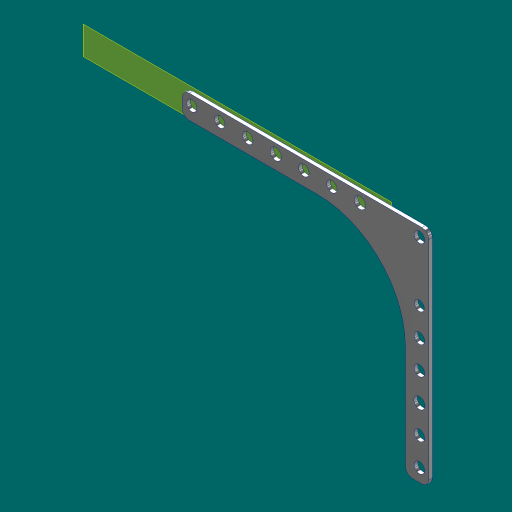
# Autodesk Inventor part: UnderGusset
Saved by Autodesk Inventor 2023.1 (Build 271208000, 208)
## iProperties
Created: 2022-11-06
Part Number: UnderGusset
Material: Aluminum 6061
Document SubType Name: Modeling
Designer: zac-h
Density: 2.7 g/cm^3
Appearance: Aluminum - Flat
Author: zac-h
Autodesk Inventor part; units mm, degrees
ref_plane "YZ Plane" through (0, 0, 0) normal (1, 0, 0) x (0, 1, 0)
ref_plane "XZ Plane" through (0, 0, 0) normal (0, 1, 0) x (-1, 0, 0)
ref_plane "XY Plane" through (0, 0, 0) normal (0, 0, 1) x (1, 0, 0)
ref_plane "Work Plane1" through (0, 0, 0) normal (0, 0, 1) x (1, 0, 0)
sketch "Sketch1" plane through (0, 0, 0) normal (0, 0, 1) x (1, 0, 0)
  line L0 (468.9048, -89.2586) -> (468.9048, 5.0009) projected
  arc A0 (468.9048, 5.0009) -> (465.7298, 8.1759) centre (465.7298, 5.0009) ccw projected
  line L1 (465.7298, 8.1759) -> (360.311, 8.1759) projected
  line L2 (458.2368, -92.4336) -> (458.2368, -2.4921)
  line L3 (458.2368, -2.4921) -> (357.136, -2.4921)
  arc A1 (360.311, 8.1759) -> (357.136, 5.0009) centre (360.311, 5.0009) ccw projected
  line L4 (357.136, 5.0009) -> (357.136, -89.2586) projected
  arc A2 (357.136, -89.2586) -> (360.311, -92.4336) centre (360.311, -89.2586) ccw projected
  line L5 (360.311, -92.4336) -> (465.7298, -92.4336) projected
  arc A3 (465.7298, -92.4336) -> (468.9048, -89.2586) centre (465.7298, -89.2586) ccw projected
  line L6 (468.9048, -89.2586) -> (468.9048, 5.0009) projected
  arc A4 (468.9048, 5.0009) -> (465.7298, 8.1759) centre (465.7298, 5.0009) ccw projected
  line L7 (465.7298, 8.1759) -> (360.311, 8.1759) projected
  circle A5 centre (437.65, 3.8619) radius 2.5844 projected
  circle A6 centre (372.6092, -23.0789) radius 2.5844 projected
  circle A7 centre (399.55, -88.1196) radius 2.5844 projected
  circle A8 centre (464.5908, -61.1789) radius 2.5844 projected
  circle A9 centre (372.6092, -88.1196) radius 2.413 projected
  circle A10 centre (412.25, 3.8619) radius 2.413 projected
  circle A11 centre (464.5908, -73.8789) radius 2.413 projected
  circle A12 centre (464.5908, -48.4789) radius 2.413 projected
  circle A13 centre (464.5908, -35.7789) radius 2.413 projected
  circle A14 centre (374.15, 3.8619) radius 2.413 projected
  circle A15 centre (386.85, 3.8619) radius 2.413 projected
  arc A16 (365.5823, -19.7251) -> (365.5823, -17.8759) centre (362.2803, -18.8005) ccw projected
  line L8 (365.5823, -19.7251) -> (365.5823, -22.1025) projected
  line L9 (365.5823, -22.1025) -> (363.2049, -22.1025) projected
  arc A17 (361.3557, -22.1025) -> (363.2049, -22.1025) centre (362.2803, -18.8005) ccw projected
  line L10 (361.3557, -22.1025) -> (358.9783, -22.1025) projected
  line L11 (358.9783, -22.1025) -> (358.9783, -19.7251) projected
  arc A18 (358.9783, -17.8759) -> (358.9783, -19.7251) centre (362.2803, -18.8005) ccw projected
  line L12 (358.9783, -17.8759) -> (358.9783, -15.4985) projected
  line L13 (358.9783, -15.4985) -> (361.3557, -15.4985) projected
  arc A19 (363.2049, -15.4985) -> (361.3557, -15.4985) centre (362.2803, -18.8005) ccw projected
  line L14 (363.2049, -15.4985) -> (365.5823, -15.4985) projected
  line L15 (365.5823, -15.4985) -> (365.5823, -17.8759) projected
  circle A20 centre (424.95, 3.8619) radius 2.413 projected
  arc A21 (358.9783, -64.5327) -> (358.9783, -66.3818) centre (362.2803, -65.4572) ccw projected
  line L16 (358.9783, -64.5327) -> (358.9783, -62.1552) projected
  line L17 (358.9783, -62.1552) -> (361.3557, -62.1552) projected
  arc A22 (363.2049, -62.1552) -> (361.3557, -62.1552) centre (362.2803, -65.4572) ccw projected
  line L18 (363.2049, -62.1552) -> (365.5823, -62.1552) projected
  line L19 (365.5823, -62.1552) -> (365.5823, -64.5327) projected
  arc A23 (365.5823, -66.3818) -> (365.5823, -64.5327) centre (362.2803, -65.4572) ccw projected
  line L20 (365.5823, -66.3818) -> (365.5823, -68.7592) projected
  line L21 (365.5823, -68.7592) -> (363.2049, -68.7592) projected
  arc A24 (361.3557, -68.7592) -> (363.2049, -68.7592) centre (362.2803, -65.4572) ccw projected
  line L22 (361.3557, -68.7592) -> (358.9783, -68.7592) projected
  line L23 (358.9783, -68.7592) -> (358.9783, -66.3818) projected
  circle A25 centre (464.5908, -86.5789) radius 2.413 projected
  circle A26 centre (464.5908, -23.0789) radius 1.9844 projected
  circle A27 centre (464.5908, 3.8619) radius 2.413 projected
  circle A28 centre (361.45, 3.8619) radius 2.413 projected
  circle A29 centre (418.6, -42.1289) radius 36.6 projected
  circle A30 centre (437.65, -88.1196) radius 2.5844 projected
  circle A31 centre (372.6092, -61.1789) radius 2.5844 projected
  circle A32 centre (399.55, 3.8619) radius 2.5844 projected
  circle A33 centre (418.6, -42.1289) radius 39.6368
  circle A34 centre (464.5908, 3.8619) radius 2.2479
  circle A35 centre (464.5908, -23.0789) radius 2.2479
  circle A36 centre (464.5908, -35.7789) radius 2.2479
  circle A37 centre (464.5908, -48.4789) radius 2.2479
  circle A38 centre (464.5908, -61.1789) radius 2.2479
  circle A39 centre (464.5908, -73.8789) radius 2.2479
  circle A40 centre (464.5908, -86.5789) radius 2.2479
  circle A41 centre (437.65, 3.8619) radius 2.2479
  circle A42 centre (424.95, 3.8619) radius 2.2479
  circle A43 centre (412.25, 3.8619) radius 2.2479
  circle A44 centre (399.55, 3.8619) radius 2.2479
  circle A45 centre (386.85, 3.8619) radius 2.2479
  circle A46 centre (374.15, 3.8619) radius 2.2479
  circle A47 centre (361.45, 3.8619) radius 2.2479
  point P0 (0, 0)
  point P1 (418.6, -2.4921)
  point P2 (458.2368, -42.1289)
  dimension "d0" = 10.668
  dimension "d2" = 4.4958
  dimension "d5" = 12.7
  dimension "d10" = 4.4958
  dimension "d13" = 12.7
  constraints: 15 centre point, 4 coincident, 4 end point, 2 point on line, 1 equal radius, 1 horizontal, 1 perpendicular, 1 tangent, 1 vertical, 23 other
  measures "d0" distance between parallel lines of L0 L2
  measures "d2" diameter of A34
  measures "d5" distance of A35.centre A36.centre
  measures "d10" diameter of A41
  measures "d13" distance of A41.centre A42.centre
extrude "Extrusion1" add sketch "Sketch1" along normal blind 1.5875 contours A3 L5 L2 L3 L4 A1 L1 A0 L0 | A33 L3 L2
fillet "Fillet1" radius 3.175 2 edges at (458.2368, -92.4336, 0.7938) (357.136, -2.4921, 0.7938)
body "Solid1"
